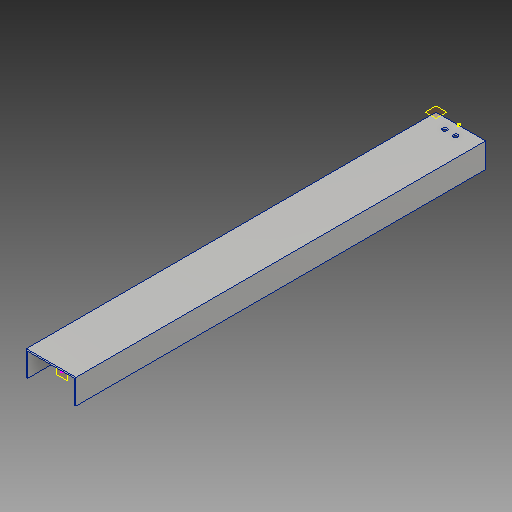
# Autodesk Inventor part: 412
Saved by Autodesk Inventor 2017 (Build 210142000, 142)
## iProperties
Created: 2018-01-12
Part Number: 412
Material: Aluminum 6061
Document SubType Name: Modeling
Designer: S332725563
Density: 2.7 g/cm^3
Appearance: Aluminum - Flat
Author: S332725563
Autodesk Inventor part; units mm, degrees
ref_plane "YZ Plane" through (0, 0, 0) normal (1, 0, 0) x (0, 1, 0)
ref_plane "XZ Plane" through (0, 0, 0) normal (0, 1, 0) x (-1, 0, 0)
ref_plane "XY Plane" through (0, 0, 0) normal (0, 0, 1) x (1, 0, 0)
sketch "Sketch1" plane through (0, 0, 0) normal (0, 0, 1) x (1, 0, 0)
  line L0 (-46.9137, 29.2863) -> (54.6863, 29.2863)
  line L1 (54.6863, 29.2863) -> (54.6863, -21.5137)
  line L2 (54.6863, -21.5137) -> (-46.9137, -21.5137)
  line L3 (-46.9137, -21.5137) -> (-46.9137, 29.2863)
  line L4 (51.5113, 26.1113) -> (-43.7387, 26.1113)
  line L5 (-43.7387, 26.1113) -> (-43.7387, -18.3387)
  line L6 (-43.7387, -18.3387) -> (51.5113, -18.3387)
  line L7 (51.5113, -18.3387) -> (51.5113, 26.1113)
  line L8 (-43.7387, -18.3387) -> (-43.7387, -21.5137)
  line L9 (51.5113, -18.3387) -> (51.5113, -21.5137)
  point P0 (0, 0)
  dimension "d0" = 50.8
  dimension "d1" = 101.6
  dimension "d4" = 3.175
  constraints: 20 end point, 4 parallel, 4 perpendicular, 2 point on line, 1 horizontal, 3 other
  measures "d0" distance of L2.end L0.start
  measures "d1" distance of L0.start L0.end
  measures "d4" distance between parallel lines of L0 L4
ref_plane "Work Plane1" through (-46.9137, 29.2863, 0) normal (0, 1, 0) x (1, 0, 0)
sketch "Sketch2" plane through (-46.9137, 29.2863, 0) normal (0, 1, 0) x (1, 0, 0)
  point P0 (46.9137, 0)
ref_plane "Work Plane2" through (0, 0, 812.8) normal (0, 0, 1) x (1, 0, 0)
sketch "Sketch3" plane through (0, 0, 812.8) normal (0, 0, 1) x (1, 0, 0)
  point P0 (0, 0)
extrude "Extrusion3" add sketch "Sketch1" along normal blind 838.2 contours L0 L1 L2 L9 L7 L4 L5 L8 L3
sketch "Sketch4" plane through (-46.9137, 29.2863, 0) normal (0, 1, 0) x (1, 0, 0)
  point P0 (46.9137, 0)
sketch "Sketch5" plane through (-46.9137, 29.2863, 0) normal (0, 1, 0) x (1, 0, 0)
  circle A0 centre (62.0522, -21.59) radius 4.826
  line L0 (101.6, 0) -> (0, 0) projected
  circle A1 centre (39.5478, -21.59) radius 4.826
  line L1 (101.6, 0) -> (101.6, -838.2) projected
  point P0 (46.9137, 0)
  dimension "d9" = 9.652
  dimension "d12" = 22.5044
  dimension "d13" = 21.59
  dimension "d17" = 39.5478
  constraints: 2 centre point, 1 equal radius, 1 horizontal alignment
  measures "d9" diameter of A0
  measures "d12" distance of A1.centre A0.centre
  measures "d13" distance from line of L0 A0.centre
  measures "d17" distance from line of L1 A0.centre
extrude "Extrusion4" cut sketch "Sketch5" against normal through all
body "Solid3"
